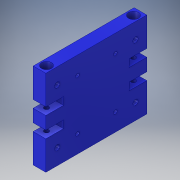
# Autodesk Inventor part: КВ33.044.501 - Каретка оси Y
Saved by Autodesk Inventor 2019 (Build 230136000, 136)
## iProperties
Created: 2019-07-21
Part Number: КВ33.044.501 - Каретка оси Y
Material: Пластик АБС
Document SubType Name: Modeling
Designer: Петров Иван
Density: 1.06 g/cm^3
Appearance: Синий — малярная краска — глянцевая
Author: Петров Иван
Autodesk Inventor part; units mm, degrees
ref_plane "YZ Plane" through (0, 0, 0) normal (1, 0, 0) x (0, 1, 0)
ref_plane "XZ Plane" through (0, 0, 0) normal (0, 1, 0) x (-1, 0, 0)
ref_plane "XY Plane" through (0, 0, 0) normal (0, 0, 1) x (1, 0, 0)
sketch "Эскиз1" plane through (0, 0, 0) normal (1, 0, 0) x (0, 1, 0)
  line L0 (-34, 40) -> (34, 40)
  line L1 (34, 40) -> (34, -40)
  line L2 (34, -40) -> (-34, -40)
  line L3 (-34, -40) -> (-34, 40)
  line L4 (-34, 40) -> (34, -40) construction
  line L5 (34, 40) -> (-34, -40) construction
  line L6 (0, 0) -> (0, 31)
  line L7 (0, 31) -> (21.48, 31)
  line L8 (0, 31) -> (-21.48, 31)
  line L9 (0, 0) -> (0, -31)
  line L10 (0, -31) -> (21.48, -31)
  line L11 (0, -31) -> (-21.48, -31)
  circle A0 centre (21.48, 31) radius 2.1
  circle A1 centre (-21.48, 31) radius 2.1
  circle A2 centre (21.48, -31) radius 2.1
  circle A3 centre (-21.48, -31) radius 2.1
  dimension "d0" = 68
  dimension "d1" = 80
  dimension "d2" = 21.48
  dimension "d3" = 21.48
  dimension "d4" = 31
  dimension "d5" = 31
  dimension "d6" = 21.48
  dimension "d7" = 21.48
  dimension "d8" = 4.2
  dimension "d9" = 4.2
  dimension "d10" = 4.2
  dimension "d11" = 4.2
  constraints: 24 end point, 4 centre point, 4 coincident, 3 horizontal, 3 perpendicular, 2 midpoint, 2 parallel, 2 vertical
  measures "d0" distance of L1.end L2.end
  measures "d1" distance of L0.end L1.end
  measures "d2" distance of L6.end L7.end
  measures "d3" distance of L6.end L8.end
  measures "d4" distance of L6.start L6.end
  measures "d5" distance of L6.start L9.end
  measures "d6" distance of L9.end L10.end
  measures "d7" distance of L9.end L11.end
  measures "d8" diameter of A0
  measures "d9" diameter of A1
  measures "d10" diameter of A2
  measures "d11" diameter of A3
extrude "Выдавливание1" add sketch "Эскиз1" along normal blind 10
sketch "Эскиз2" plane through (10, 0, 0) normal (1, 0, 0) x (0, 0, -1)
  line L0 (-40, 34) -> (-40, -34) projected
  line L1 (-40, 0) -> (-40, 5)
  line L2 (-40, 0) -> (-26, 0)
  line L3 (-26, 0) -> (-26, 11)
  line L4 (-40, 5) -> (-26, 5)
  line L5 (-26, 5) -> (-26, 11)
  line L6 (-26, 11) -> (-40, 11)
  line L7 (-40, 11) -> (-40, 5)
  line L8 (-40, 0) -> (-40, -5)
  line L9 (-26, 0) -> (-26, -11)
  line L10 (-40, -5) -> (-26, -5)
  line L11 (-26, -5) -> (-26, -11)
  line L12 (-26, -11) -> (-40, -11)
  line L13 (-40, -11) -> (-40, -5)
  line L14 (40, -34) -> (40, 34) projected
  line L15 (40, 0) -> (40, 5)
  line L16 (40, 0) -> (26, 0)
  line L17 (26, 0) -> (26, 11)
  line L18 (26, 11) -> (40, 11)
  line L19 (40, 11) -> (40, 5)
  line L20 (40, 5) -> (26, 5)
  line L21 (26, 5) -> (26, 11)
  line L22 (26, 0) -> (26, -11)
  line L23 (40, 0) -> (40, -5)
  line L24 (26, -11) -> (40, -11)
  line L25 (40, -11) -> (40, -5)
  line L26 (40, -5) -> (26, -5)
  line L27 (26, -5) -> (26, -11)
  point P0 (0, 0)
  dimension "d14" = 5
  dimension "d15" = 14
  dimension "d16" = 11
  dimension "d17" = 5
  dimension "d18" = 11
  dimension "d19" = 5
  dimension "d20" = 14
  dimension "d21" = 11
  dimension "d22" = 11
  dimension "d23" = 5
  constraints: 52 end point, 8 parallel, 7 perpendicular, 5 horizontal, 4 point on line, 2 midpoint, 2 vertical
  measures "d14" distance of L1.start L1.end
  measures "d15" distance of L1.start L2.end
  measures "d16" distance of L2.end L3.end
  measures "d17" distance of L1.start L8.end
  measures "d18" distance of L2.end L9.end
  measures "d19" distance of L15.start L15.end
  measures "d20" distance of L15.start L16.end
  measures "d21" distance of L16.end L17.end
  measures "d22" distance of L16.end L22.end
  measures "d23" distance of L15.start L23.end
extrude "Выдавливание2" cut sketch "Эскиз2" against normal blind 10 contours L6 L3 L4 L0 | L10 L9 L12 L0 | L24 L22 L26 L14 | L20 L17 L18 L14
sketch "Эскиз3" plane through (0, 34, 40) normal (0, 1, 0) x (1, 0, 0)
  line L0 (0, 0) -> (10, 0) projected
  line L1 (5, 0) -> (5, 11.1)
  line L2 (0, 11.1) -> (10, 11.1) projected
  circle A0 centre (5, 5.55) radius 1.8
  line L3 (0, 80) -> (10, 80) projected
  line L4 (5, 80) -> (5, 68.9)
  line L5 (0, 68.9) -> (10, 68.9) projected
  circle A1 centre (5, 74.45) radius 1.8
  point P0 (0, 40)
  dimension "d26" = 3.6
  dimension "d29" = 3.6
  constraints: 6 midpoint, 4 end point, 2 centre point
  measures "d26" diameter of A0
  measures "d29" diameter of A1
extrude "Выдавливание3" cut sketch "Эскиз3" against normal through all
sketch "Эскиз4" plane through (0, 34, 40) normal (0, 1, 0) x (1, 0, 0)
  circle A0 centre (5, 5.55) radius 1.8 projected
  circle A1 centre (5, 5.55) radius 4
  circle A2 centre (5, 74.45) radius 1.8 projected
  circle A3 centre (5, 74.45) radius 4
  point P0 (0, 40)
  dimension "d30" = 8
  dimension "d31" = 8
  constraints: 2 centre point, 2 coincident
  measures "d30" diameter of A1
  measures "d31" diameter of A3
extrude "Выдавливание4" cut sketch "Эскиз4" against normal blind 10
sketch "Эскиз5" plane through (10, 0, 0) normal (1, 0, 0) x (0, 0, -1)
  line L0 (0, 0) -> (0, 18)
  line L1 (0, 18) -> (0, 20)
  line L2 (0, 20) -> (-15, 20)
  line L3 (-15, 20) -> (15, 20)
  circle A0 centre (-15, 20) radius 1.5
  circle A1 centre (15, 20) radius 1.5
  line L4 (0, 0) -> (6.6954, 0)
  line L5 (0, -18) -> (0, -20)
  line L6 (0, -20) -> (-15, -20)
  line L7 (-15, -20) -> (15, -20)
  circle A2 centre (-15, -20) radius 1.5
  circle A3 centre (15, -20) radius 1.5
  dimension "d34" = 18
  dimension "d35" = 2
  dimension "d36" = 15
  dimension "d37" = 30
  dimension "d38" = 3
  dimension "d39" = 3
  constraints: 16 end point, 6 symmetric about line, 4 centre point, 4 coincident, 3 point on line, 2 horizontal, 1 vertical, 2 other
  measures "d34" distance of L0.start L0.end
  measures "d35" distance of L0.end L1.end
  measures "d36" distance of L1.end L2.end
  measures "d37" distance of L2.end L3.end
  measures "d38" diameter of A0
  measures "d39" diameter of A1
extrude "Выдавливание5" cut sketch "Эскиз5" against normal blind 10
equation "\"d3\" = d2"
equation "\"d5\" = d4"
equation "\"d6\" = d2"
equation "\"d7\" = d2"
equation "\"d9\" = d8"
equation "\"d10\" = d8"
equation "\"d11\" = d8"
equation "\"d17\" = d14"
equation "\"d18\" = d16"
equation "\"d19\" = d14"
equation "\"d21\" = d16"
equation "\"d22\" = d16"
equation "\"d23\" = d14"
